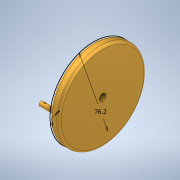
# Autodesk Inventor part: extension circle
Saved by Autodesk Inventor 2022 (Build 260153070, 153G)
## iProperties
Created: 2021-07-02
Part Number: extension circle
Material: Brass, Soft Yellow
Document SubType Name: Modeling
Designer: AKASH ARYAN
Density: 8.47 g/cm^3
Appearance: Brass - Satin
Author: AKASH ARYAN
Autodesk Inventor part; units mm, degrees
ref_plane "YZ Plane" through (0, 0, 0) normal (1, 0, 0) x (0, 1, 0)
ref_plane "XZ Plane" through (0, 0, 0) normal (0, 1, 0) x (-1, 0, 0)
ref_plane "XY Plane" through (0, 0, 0) normal (0, 0, 1) x (1, 0, 0)
sketch "Sketch1" plane through (0, 0, 0) normal (1, 0, 0) x (0, 1, 0)
  circle A0 centre (0, 0) radius 38.1
  circle A1 centre (0, 31.6517) radius 2
  dimension "d0" = 76.2
  dimension "d14" = 4
  constraints: 2 centre point, 1 coincident
  measures "d0" diameter of A0
  measures "d14" diameter of A1
extrude "Extrusion1" add sketch "Sketch1" along normal blind 8 contours A0 | A1
sketch "Sketch2" plane through (8, 0, 0) normal (1, 0, 0) x (0, 0, -1)
  circle A0 centre (0, 0) radius 3
  dimension "d3" = 6
  constraints: 1 centre point, 1 coincident
  measures "d3" diameter of A0
extrude "Extrusion2" cut sketch "Sketch2" against normal through all
fillet "Fillet1" radius 2 2 edges at (8, -38.1, 0) (0, -38.1, 0)
sketch "Sketch4" plane through (8, 0, 0) normal (1, 0, 0) x (0, 0, -1)
  point P0 (0, 0)
sketch "Sketch7" plane through (8, 0, 0) normal (1, 0, 0) x (0, 0, -1)
  point P0 (0, 0)
extrude "Extrusion5" add sketch "Sketch1" against normal blind 14 contours A1
sketch "Sketch8" plane through (0, 0, 0) normal (0, 1, 0) x (-1, 0, 0)
  circle A0 centre (11, 31.2419) radius 1
  line L0 (14, 29.6517) -> (14, 33.6517) projected
  point P0 (0, 0)
  dimension "d17" = 2
  dimension "d18" = 3
  constraints: 1 centre point
  measures "d17" diameter of A0
  measures "d18" distance from line of L0 A0.centre
extrude "Extrusion6" cut sketch "Sketch8" along normal mid plane 14
body "Solid1"
